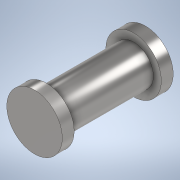
# Autodesk Inventor part: Nit tarczy długi
Saved by Autodesk Inventor 2022 (Build 260153000, 153)
## iProperties
Created: 2021-06-26
Part Number: Nit tarczy długi
Material: Stal, węglowa
Document SubType Name: Modeling
Designer: Matik
Density: 7.85 g/cm^3
Appearance: Częściowo polerowany
Author: Matik
Autodesk Inventor part; units mm, degrees
ref_plane "YZ Plane" through (0, 0, 0) normal (1, 0, 0) x (0, 1, 0)
ref_plane "XZ Plane" through (0, 0, 0) normal (0, 1, 0) x (-1, 0, 0)
ref_plane "Płaszczyzna konstrukcyjna1" through (0, 0, 0) normal (0, 0, 1) x (1, 0, 0)
sketch "Szkic1" plane through (0, 0, 0) normal (0, 0, 1) x (1, 0, 0)
  circle A0 centre (-13, -22.5167) radius 2.5 projected
  circle A1 centre (-13, -22.5167) radius 2.5
  point P0 (0, 0)
  constraints: 1 centre point, 1 coincident, 1 concentric
extrude "Wyciągnięcie proste1" add sketch "Szkic1" against normal blind 11
sketch "Szkic2" plane through (-13, -22.5167, -11) normal (0, 0, -1) x (-1, 0, 0)
  circle A0 centre (0, 0) radius 2.5 projected
  circle A1 centre (0, 0) radius 3.5
  point P0 (-13, 22.5167)
  dimension "d2" = 7
  constraints: 1 centre point, 1 coincident
  measures "d2" diameter of A1
extrude "Wyciągnięcie proste2" add sketch "Szkic2" along normal blind 1.5 contours A0 | A1
sketch "Szkic3" plane through (-13, -22.5167, 0) normal (0, 0, 1) x (1, 0, 0)
  circle A0 centre (0, 0) radius 3.5
  point P0 (13, 22.5167)
  dimension "d5" = 7
  constraints: 1 centre point
  measures "d5" diameter of A0
extrude "Wyciągnięcie proste3" add sketch "Szkic3" along normal blind 1.5
